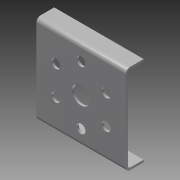
# Autodesk Inventor part: Plate (Front)
Saved by Autodesk Inventor 2014 (Build 180170000, 170)
## iProperties
Created: 2014-01-12
Part Number: Plate (Front)
Material: Steel
Document SubType Name: Sheet Metal
Designer: Andrew Toennies
Mass: 284.154 g
Surface Area: 250.82 cm^2
Volume: 36.1979 cm^3
Density: 7.85 g/cm^3
Sheet Metal Rule: Default
Appearance: Steel
Author: Andrew Toennies
Autodesk Inventor part; units mm, degrees
ref_plane "YZ Plane" through (0, 0, 0) normal (1, 0, 0) x (0, 1, 0)
ref_plane "XZ Plane" through (0, 0, 0) normal (0, 1, 0) x (-1, 0, 0)
ref_plane "XY Plane" through (0, 0, 0) normal (0, 0, 1) x (1, 0, 0)
sketch "Sketch3" plane through (0, 0, 0) normal (0, 0, -1) x (-1, 0, 0)
  circle A0 centre (0, 0) radius 63.5
  line L0 (-63.5, 63.5) -> (63.5, 63.5)
  line L1 (63.5, 63.5) -> (63.5, -63.5)
  line L2 (63.5, -63.5) -> (-63.5, -63.5)
  line L3 (-63.5, -63.5) -> (-63.5, 63.5)
sketch "Sketch1" plane through (0, 0, 0) normal (0, 0, 1) x (1, 0, 0)
  circle A0 centre (0, 0) radius 63.5
  circle A1 centre (0, 0) radius 12.7
  circle A2 centre (0, 41.275) radius 6.35
  line L0 (0, 0) -> (0, 41.275) construction
  line L1 (0, 41.275) -> (0, 57.9438) construction
  line L2 (-16.6688, 41.275) -> (16.6688, 41.275) construction
  circle A3 centre (-35.7452, 20.6375) radius 6.35
  circle A4 centre (-35.7452, -20.6375) radius 6.35
  circle A5 centre (0, -41.275) radius 6.35
  circle A6 centre (35.7452, -20.6375) radius 6.35
  circle A7 centre (35.7452, 20.6375) radius 6.35
  dimension "d0" = 127
  dimension "d1" = 25.4
  dimension "d2" = 12.7
  dimension "d3" = 41.275
  dimension "d22" = 360
  constraints: 8 centre point, 6 end point, 3 coincident, 2 vertical, 1 midpoint, 1 perpendicular, 13 other
  measures "d0" diameter of A0
  measures "d1" diameter of A1
  measures "d2" diameter of A2
  measures "d3" distance of L0.start L0.end
extrude "Plate2" add sketch "Sketch1" along normal blind 3.175
sheet face with bend "Face3" sketch "Sketch3" thickness 3.175 toward (0, 0, 1) bend radius 3.175 relief straight relief width 3.175 relief depth 1.5875 contours L1 L2 A0 | A0 L0 L1 | A0 L3 L0 | L2 L3 A0
bend "Bend1"
sketch "Sketch4" plane through (-63.5, -60.325, 3.175) normal (0, -1, 0) x (1, 0, 0)
  line L0 (127, 0) -> (0, 0)
  line L1 (0, 0) -> (0, -25.4)
  line L2 (0, -25.4) -> (127, -25.4)
  line L3 (127, -25.4) -> (127, 0)
  constraints: 6 end point, 1 horizontal, 1 perpendicular, 1 vertical
edge flange "Flange1" height 25.4 angle 90 thickness 3.175 bend radius 3.175 thickness toward (0, -1, 0) relief straight relief width 3.175 relief depth 1.5875 corner gap 3.175 corner form 0 edges at (0, -63.5, 0) (0, 63.5, 0) wall of the first edge with corners at (63.5, -60.325, 3.175) (-63.5, -60.325, 3.175) (-63.5, -60.325, -22.225) (63.5, -60.325, -22.225)
bend "Bend2"
corner "Corner1"
equation "\"d24\" = BendRadius"
equation "\"d25\" = BendReliefWidth"
equation "\"d27\" = MinimumRemnant"
equation "\"d26\" = BendReliefDepth"
equation "\"d28\" = BendRadius"
equation "\"d29\" = BendReliefWidth"
equation "\"d30\" = BendReliefDepth"
equation "\"d31\" = MinimumRemnant"
equation "\"d32\" = BendRadius"
equation "\"d35\" = BendRadius"
equation "\"d36\" = CornerReliefSize"
equation "\"d37\" = GapSize"
equation "\"d38\" = JacobiRadiusSize"
equation "\"BendRadius\" = Thickness"
equation "\"BendReliefWidth\" = Thickness"
equation "\"BendReliefDepth\" = 0.5 * Thickness"
equation "\"CornerReliefSize\" = 4 * Thickness"
equation "\"MinimumRemnant\" = 2 * Thickness"
equation "\"TransitionRadius\" = BendRadius"
equation "\"JacobiRadiusSize\" = BendRadius"
equation "\"GapSize\" = Thickness"
equation "\"d8\" = BendRadius"
equation "\"d19\" = BendRadius"
equation "\"Thickness\" = 3.175"
body "Solid2"
